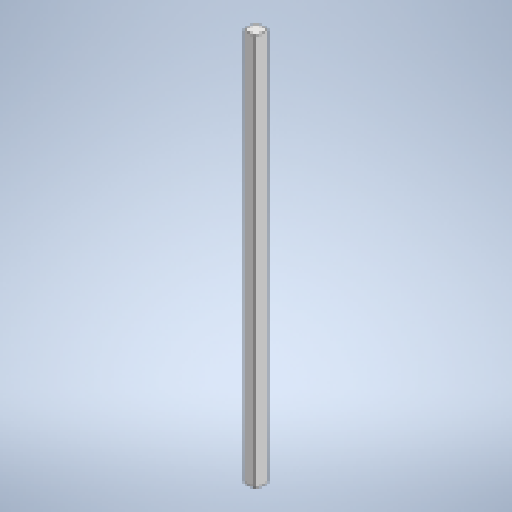
# Autodesk Inventor part: Barra inversa
Saved by Autodesk Inventor 2024 (Build 280153000, 153)
## iProperties
Created: 2023-07-03
Part Number: Barra inversa
Material: Genérico
Document SubType Name: Modeling
Designer: sergi
Density: 1 g/cm^3
Appearance: Valor por defecto
Author: sergi
Autodesk Inventor part; units mm, degrees
ref_plane "YZ Plane" through (0, 0, 0) normal (1, 0, 0) x (0, 1, 0)
ref_plane "XZ Plane" through (0, 0, 0) normal (0, 1, 0) x (-1, 0, 0)
ref_plane "XY Plane" through (0, 0, 0) normal (0, 0, 1) x (1, 0, 0)
ref_plane "Plano de trabajo1" through (-15, 0, -15) normal (0, -1, 0) x (1, 0, 0)
sketch "Boceto2" plane through (-15, 0, -15) normal (0, -1, 0) x (1, 0, 0)
  line L0 (566, 15) -> (1911, 15) projected
  line L1 (566, 536) -> (566, 15) projected
  line L2 (1911, 536) -> (566, 536) projected
  line L3 (1911, 15) -> (1911, 536) projected
  line L4 (536, 1414) -> (15, 1414) projected
  line L5 (536, 15) -> (536, 1414) projected
  line L6 (15, 15) -> (536, 15) projected
  line L7 (15, 1414) -> (15, 15) projected
  line L8 (-15, 1444) -> (566, 1444) projected
  line L9 (-15, -15) -> (-15, 1444) projected
  line L10 (1941, -15) -> (-15, -15) projected
  line L11 (1941, 566) -> (1941, -15) projected
  line L12 (566, 566) -> (1941, 566) projected
  line L13 (566, 1444) -> (566, 566) projected
  line L14 (566, 566) -> (566, 544.7868)
  line L15 (6.2132, -15) -> (15, -15)
  line L16 (544.7868, 566) -> (-15, 6.2132)
  line L17 (566, 544.7868) -> (6.2132, -15)
  line L18 (566, 566) -> (544.7868, 566)
  line L19 (-15, 6.2132) -> (-15, -15)
  line L20 (6.2132, -15) -> (-15, -15)
  point P0 (6.2132, -15)
  dimension "d4" = 30
  dimension "d6" = 30
  constraints: 14 end point, 3 point on line, 1 collinear, 1 parallel, 1 vertical
  measures "d4" distance of L9.start L15.end
  measures "d6" distance between parallel lines of L16 L17
extrude "Extrusión2" add sketch "Boceto2" against normal blind 770 contours L16 L18 L14 L17 L5 | L5 L17 L6 L7 L16 | L7 L6 L17 L10 L9 L16
sketch "Boceto3" plane through (-15, 0, -15) normal (0, -1, 0) x (1, 0, 0)
  line L0 (566, 544.7868) -> (566, 566) projected
  line L1 (566, 566) -> (544.7868, 566) projected
  line L2 (544.7868, 566) -> (-15, 6.2132) projected
  line L3 (-15, 6.2132) -> (-15, -15) projected
  line L4 (-15, -15) -> (6.2132, -15) projected
  line L5 (6.2132, -15) -> (566, 544.7868) projected
  line L6 (-15, -15) -> (15, -15)
  line L7 (15, -15) -> (15, 15)
  line L8 (15, 15) -> (-15, 15)
  line L9 (-15, 15) -> (-15, -15)
  point P0 (-6.2132, 15)
  point P1 (15, -6.2132)
  dimension "d9" = 30
  dimension "d10" = 30
  constraints: 8 end point, 2 parallel, 1 horizontal, 1 perpendicular
  measures "d9" distance of L8.end L7.end
  measures "d10" distance of L7.end L6.end
extrude "Extrusión3" cut sketch "Boceto3" against normal blind 770 contours L5 L4 L3 L2 L8 L7
sketch "Boceto4" plane through (551, 0, 529.7868) normal (0.7071, 0, -0.7071) x (-0.7071, 0, -0.7071)
  line L0 (764.2317, 0) -> (764.2317, 770) projected
  line L1 (764.2317, 0) -> (764.2317, 770)
  line L2 (779.2317, 0) -> (764.2317, 0) projected
  line L3 (-9.9264, 770) -> (764.2317, 0)
  line L4 (13.656, 788.8569) -> (806.7728, 0)
  line L5 (779.2317, 0) -> (779.2317, 770) projected
  line L6 (0, 770) -> (779.2317, 770) projected
  line L7 (0, 0) -> (0, 770) projected
  line L8 (779.2317, 0) -> (0, 0) projected
  line L9 (0, 0) -> (-15, 0) projected
  line L10 (0, 0) -> (0, 770) projected
  line L11 (-15, 770) -> (0, 770) projected
  line L12 (-15, 0) -> (-15, 770) projected
  line L13 (779.2317, 0) -> (779.2317, 770) projected
  line L14 (0, 770) -> (779.2317, 770) projected
  line L15 (0, 0) -> (0, 770) projected
  line L16 (779.2317, 0) -> (0, 0) projected
  point P0 (32.6148, 770)
  point P1 (779.2317, 27.3932)
  point P2 (764.2317, 0)
  dimension "d13" = 30
  constraints: 6 end point, 2 point on line, 1 collinear, 1 parallel
  measures "d13" distance between parallel lines of L3 L4
extrude "Extrusión4" cut sketch "Boceto4" against normal blind 770 contours L8 L7 L3 | L4 L6 L0 | L0 L6 L5 L4 | L7 L9 L12 L11 L3
